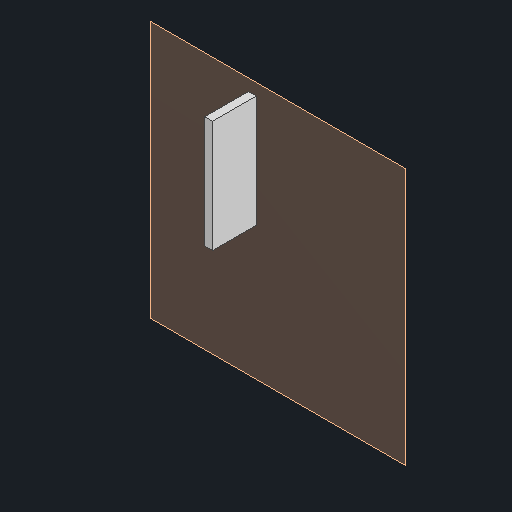
# Autodesk Inventor part: right_gear_holder
Saved by Autodesk Inventor 2023 (Build 270158000, 158)
## iProperties
Created: 2024-04-23
Part Number: right_gear_holder
Material: Generic
Document SubType Name: Modeling
Designer: szymo
Density: 1 g/cm^3
Appearance: Default
Author: szymo
Autodesk Inventor part; units mm, degrees
ref_plane "YZ Plane" through (0, 0, 0) normal (1, 0, 0) x (0, 1, 0)
ref_plane "XZ Plane" through (0, 0, 0) normal (0, 1, 0) x (-1, 0, 0)
ref_plane "XY Plane" through (0, 0, 0) normal (0, 0, 1) x (1, 0, 0)
ref_plane "Work Plane1" through (0, 0, 0) normal (0, 0, 1) x (1, 0, 0)
sketch "Sketch1" plane through (0, 0, 0) normal (0, 0, 1) x (1, 0, 0)
  line L0 (23.5, 89.5) -> (-23.5, 89.5) projected
  line L1 (-23.5, 89.5) -> (-23.5, 34.5) projected
  line L2 (-23.5, 34.5) -> (-89, 34.5) projected
  line L3 (-89, 34.5) -> (-89, -69.5) projected
  line L4 (-89, -69.5) -> (-74, -69.5) projected
  line L5 (-74, -69.5) -> (-74, -89.5) projected
  line L6 (-74, -89.5) -> (74, -89.5) projected
  line L7 (74, -89.5) -> (74, -69.5) projected
  line L8 (74, -69.5) -> (89, -69.5) projected
  line L9 (89, -69.5) -> (89, 34.5) projected
  line L10 (89, 34.5) -> (23.5, 34.5) projected
  line L11 (23.5, 34.5) -> (23.5, 89.5) projected
  line L12 (-4.5, 85.5) -> (-4.5, 34.5) projected
  line L13 (-4.5, 34.5) -> (-16.5, 34.5) projected
  line L14 (-16.5, 34.5) -> (-16.5, 85.5) projected
  line L15 (-16.5, 85.5) -> (-4.5, 85.5) projected
  line L16 (16.5, 85.5) -> (16.5, 34.5) projected
  line L17 (16.5, 34.5) -> (4.5, 34.5) projected
  line L18 (4.5, 34.5) -> (4.5, 85.5) projected
  line L19 (4.5, 85.5) -> (16.5, 85.5) projected
  line L20 (-16.5, 89.5) -> (-22.5, 89.5)
  line L21 (-22.5, 89.5) -> (-22.5, 3.75)
  line L22 (-22.5, 3.75) -> (-16.5, 3.75)
  line L23 (-16.5, 3.75) -> (-16.5, 89.5)
  line L24 (-32.2, 4.75) -> (-59.9, 4.75)
  point P0 (0, 0)
  point P1 (-16.5, 34.5)
  point P2 (-16.5, 85.5)
  dimension "d0" = 1
  dimension "d2" = 1
  constraints: 10 end point, 2 horizontal, 2 parallel, 1 collinear, 1 perpendicular, 1 point on line, 2 other
  measures "d0" distance between parallel lines of L1 L21
  measures "d2" distance between parallel lines of L24 L22
ref_plane "Work Plane2" through (-89, -40.3889, 33.5) normal (0, 0, 1) x (1, 0, 0)
extrude "Extrusion1" add sketch "Sketch1" along normal up to surface (33.5 mm away) contours L23 L14 L22 L21 L0
body "Solid1"
